Autodesk Inventor part; units mm, degrees
(part 4 of 6)
  line L1529 (-7.6457, 95.9463) -> (-7.8856, 95.9463) construction
  spline S416 degree 2 poles (-4.0547, 94.5107) (-4.2946, 94.5107) (-4.2946, 94.7506) knots 0 0 0 1 1 1
  line L1530 (-4.0547, 94.5107) -> (-4.2946, 94.5107) construction
  line L1531 (-4.2946, 94.5107) -> (-4.2946, 94.7506) construction
  spline S417 degree 2 poles (-5.0544, 95.8103) (-5.1464, 95.6784) (-5.2503, 95.6784) knots 0 0 0 1 1 1
  line L1532 (-5.0544, 95.8103) -> (-5.1464, 95.6784) construction
  line L1533 (-5.1464, 95.6784) -> (-5.2503, 95.6784) construction
  spline S418 degree 2 poles (-5.2503, 95.6784) (-5.3543, 95.6784) (-5.4463, 95.8103) knots 0 0 0 1 1 1
  line L1534 (-5.2503, 95.6784) -> (-5.3543, 95.6784) construction
  line L1535 (-5.3543, 95.6784) -> (-5.4463, 95.8103) construction
  spline S419 degree 2 poles (-6.2061, 94.7506) (-6.2061, 94.5107) (-6.446, 94.5107) knots 0 0 0 1 1 1
  line L1536 (-6.2061, 94.7506) -> (-6.2061, 94.5107) construction
  line L1537 (-6.2061, 94.5107) -> (-6.446, 94.5107) construction
  spline S420 degree 2 poles (-6.446, 94.5107) (-6.6859, 94.5107) (-6.6859, 94.7506) knots 0 0 0 1 1 1
  line L1538 (-6.446, 94.5107) -> (-6.6859, 94.5107) construction
  line L1539 (-6.6859, 94.5107) -> (-6.6859, 94.7506) construction
  line L1540 (-6.6859, 94.7506) -> (-6.6859, 97.6258)
  spline S421 degree 2 poles (-6.6859, 97.6258) (-6.6859, 97.9018) (-6.474, 97.9018) knots 0 0 0 1 1 1
  line L1541 (-6.6859, 97.6258) -> (-6.6859, 97.9018) construction
  line L1542 (-6.6859, 97.9018) -> (-6.474, 97.9018) construction
  spline S422 degree 2 poles (-6.474, 97.9018) (-6.35, 97.9018) (-6.25, 97.7618) knots 0 0 0 1 1 1
  line L1543 (-6.474, 97.9018) -> (-6.35, 97.9018) construction
  line L1544 (-6.35, 97.9018) -> (-6.25, 97.7618) construction
  spline S423 degree 2 poles (-4.2506, 97.7618) (-4.1506, 97.9018) (-4.0267, 97.9018) knots 0 0 0 1 1 1
  line L1545 (-4.2506, 97.7618) -> (-4.1506, 97.9018) construction
  line L1546 (-4.1506, 97.9018) -> (-4.0267, 97.9018) construction
  spline S424 degree 2 poles (-4.0267, 97.9018) (-3.8147, 97.9018) (-3.8147, 97.6258) knots 0 0 0 1 1 1
  line L1547 (-4.0267, 97.9018) -> (-3.8147, 97.9018) construction
  line L1548 (-3.8147, 97.9018) -> (-3.8147, 97.6258) construction
  line L1549 (-3.8147, 97.6258) -> (-3.8147, 94.7506)
  spline S425 degree 2 poles (-3.8147, 94.7506) (-3.8147, 94.5107) (-4.0547, 94.5107) knots 0 0 0 1 1 1
  line L1550 (-3.8147, 94.7506) -> (-3.8147, 94.5107) construction
  line L1551 (-3.8147, 94.5107) -> (-4.0547, 94.5107) construction
  spline S426 degree 2 poles (-0.2237, 94.5107) (-0.4637, 94.5107) (-0.4637, 94.7506) knots 0 0 0 1 1 1
  line L1552 (-0.2237, 94.5107) -> (-0.4637, 94.5107) construction
  line L1553 (-0.4637, 94.5107) -> (-0.4637, 94.7506) construction
  line L1554 (-0.4637, 94.7506) -> (-0.4637, 97.6218)
  spline S427 degree 2 poles (-0.4637, 97.6218) (-0.4637, 97.8618) (-0.2237, 97.8618) knots 0 0 0 1 1 1
  line L1555 (-0.4637, 97.6218) -> (-0.4637, 97.8618) construction
  line L1556 (-0.4637, 97.8618) -> (-0.2237, 97.8618) construction
  spline S428 degree 2 poles (-0.2237, 97.8618) (0.0162, 97.8618) (0.0162, 97.6218) knots 0 0 0 1 1 1
  line L1557 (-0.2237, 97.8618) -> (0.0162, 97.8618) construction
  line L1558 (0.0162, 97.8618) -> (0.0162, 97.6218) construction
  line L1559 (0.0162, 97.6218) -> (0.0162, 94.7506)
  spline S429 degree 2 poles (0.0162, 94.7506) (0.0162, 94.5107) (-0.2237, 94.5107) knots 0 0 0 1 1 1
  line L1560 (0.0162, 94.7506) -> (0.0162, 94.5107) construction
  line L1561 (0.0162, 94.5107) -> (-0.2237, 94.5107) construction
  spline S430 degree 2 poles (-14.794, 103.4621) (-14.4671, 103.4675) (-14.0039, 103.7345) (-13.8405, 104.1159) knots 0 0 0 1 2 2 2
  line L1562 (-14.794, 103.4621) -> (-14.4671, 103.4675) construction
  line L1563 (-14.4671, 103.4675) -> (-14.0039, 103.7345) construction
  line L1564 (-14.0039, 103.7345) -> (-13.8405, 104.1159) construction
  spline S431 degree 2 poles (-13.8405, 104.1159) (-13.7914, 104.2303) (-13.6716, 104.53) (-13.6334, 104.6444) knots 0 0 0 1 2 2 2
  line L1565 (-13.8405, 104.1159) -> (-13.7914, 104.2303) construction
  line L1566 (-13.7914, 104.2303) -> (-13.6716, 104.53) construction
  line L1567 (-13.6716, 104.53) -> (-13.6334, 104.6444) construction
  spline S432 degree 2 poles (-13.6334, 104.6444) (-13.4373, 105.2002) (-12.7344, 105.6579) (-12.1677, 105.6579) knots 0 0 0 1 2 2 2
  line L1568 (-13.6334, 104.6444) -> (-13.4373, 105.2002) construction
  line L1569 (-13.4373, 105.2002) -> (-12.7344, 105.6579) construction
  line L1570 (-12.7344, 105.6579) -> (-12.1677, 105.6579) construction
  spline S433 degree 2 poles (-12.135, 104.9278) (-12.4892, 104.9278) (-12.8434, 104.6335) (-12.9632, 104.2412) knots 0 0 0 1 2 2 2
  line L1571 (-12.135, 104.9278) -> (-12.4892, 104.9278) construction
  line L1572 (-12.4892, 104.9278) -> (-12.8434, 104.6335) construction
  line L1573 (-12.8434, 104.6335) -> (-12.9632, 104.2412) construction
  spline S434 degree 2 poles (-12.9632, 104.2412) (-13.0886, 103.8489) (-13.4318, 103.413) (-13.6389, 103.2931) knots 0 0 0 1 2 2 2
  line L1574 (-12.9632, 104.2412) -> (-13.0886, 103.8489) construction
  line L1575 (-13.0886, 103.8489) -> (-13.4318, 103.413) construction
  line L1576 (-13.4318, 103.413) -> (-13.6389, 103.2931) construction
  spline S435 degree 2 poles (21.3473, 101.4733) (21.5271, 101.5931) (21.696, 101.9092) (21.696, 102.1598) knots 0 0 0 1 2 2 2
  line L1577 (21.3473, 101.4733) -> (21.5271, 101.5931) construction
  line L1578 (21.5271, 101.5931) -> (21.696, 101.9092) construction
  line L1579 (21.696, 101.9092) -> (21.696, 102.1598) construction
  spline S436 degree 2 poles (21.696, 102.1598) (21.696, 102.3887) (21.538, 102.7374) (21.3582, 102.8463) knots 0 0 0 1 2 2 2
  line L1580 (21.696, 102.1598) -> (21.696, 102.3887) construction
  line L1581 (21.696, 102.3887) -> (21.538, 102.7374) construction
  line L1582 (21.538, 102.7374) -> (21.3582, 102.8463) construction
  spline S437 degree 2 poles (21.3582, 102.8463) (21.1675, 102.9608) (20.688, 103.0044) (20.2412, 103.0044) knots 0 0 0 1 2 2 2
  line L1583 (21.3582, 102.8463) -> (21.1675, 102.9608) construction
  line L1584 (21.1675, 102.9608) -> (20.688, 103.0044) construction
  line L1585 (20.688, 103.0044) -> (20.2412, 103.0044) construction
  spline S438 degree 2 poles (20.2194, 101.288) (20.6716, 101.288) (21.1675, 101.3643) (21.3473, 101.4733) knots 0 0 0 1 2 2 2
  line L1586 (20.2194, 101.288) -> (20.6716, 101.288) construction
  line L1587 (20.6716, 101.288) -> (21.1675, 101.3643) construction
  line L1588 (21.1675, 101.3643) -> (21.3473, 101.4733) construction
  spline S439 degree 2 poles (22.0284, 101.0265) (21.7287, 100.8031) (21.053, 100.6124) (20.5245, 100.6124) knots 0 0 0 1 2 2 2
  line L1589 (22.0284, 101.0265) -> (21.7287, 100.8031) construction
  line L1590 (21.7287, 100.8031) -> (21.053, 100.6124) construction
  line L1591 (21.053, 100.6124) -> (20.5245, 100.6124) construction
  spline S440 degree 2 poles (20.5463, 103.6909) (21.113, 103.6909) (21.7396, 103.571) (22.0502, 103.3422) knots 0 0 0 1 2 2 2
  line L1592 (20.5463, 103.6909) -> (21.113, 103.6909) construction
  line L1593 (21.113, 103.6909) -> (21.7396, 103.571) construction
  line L1594 (21.7396, 103.571) -> (22.0502, 103.3422) construction
  spline S441 degree 2 poles (22.0502, 103.3422) (22.3117, 103.1515) (22.5732, 102.5467) (22.5732, 102.1762) knots 0 0 0 1 2 2 2
  line L1595 (22.0502, 103.3422) -> (22.3117, 103.1515) construction
  line L1596 (22.3117, 103.1515) -> (22.5732, 102.5467) construction
  line L1597 (22.5732, 102.5467) -> (22.5732, 102.1762) construction
  spline S442 degree 2 poles (22.5732, 102.1762) (22.5732, 101.8111) (22.279, 101.2117) (22.0284, 101.0265) knots 0 0 0 1 2 2 2
  line L1598 (22.5732, 102.1762) -> (22.5732, 101.8111) construction
  line L1599 (22.5732, 101.8111) -> (22.279, 101.2117) construction
  line L1600 (22.279, 101.2117) -> (22.0284, 101.0265) construction
  spline S443 degree 2 poles (-15.4296, 28.4883) (-15.4296, 28.5843) (-15.2856, 28.7283) (-15.1896, 28.7283) knots 0 0 0 1 2 2 2
  line L1601 (-15.4296, 28.4883) -> (-15.4296, 28.5843) construction
  line L1602 (-15.4296, 28.5843) -> (-15.2856, 28.7283) construction
  line L1603 (-15.2856, 28.7283) -> (-15.1896, 28.7283) construction
  line L1604 (-15.1896, 28.7283) -> (-13.994, 28.7283)
  spline S444 degree 2 poles (-11.0308, 28.5323) (-10.6469, 28.7283) (-10.163, 28.7283) knots 0 0 0 1 1 1
  line L1605 (-11.0308, 28.5323) -> (-10.6469, 28.7283) construction
  line L1606 (-10.6469, 28.7283) -> (-10.163, 28.7283) construction
  spline S445 degree 2 poles (-10.163, 28.7283) (-9.4432, 28.7283) (-8.8754, 28.3244) knots 0 0 0 1 1 1
  line L1607 (-10.163, 28.7283) -> (-9.4432, 28.7283) construction
  line L1608 (-9.4432, 28.7283) -> (-8.8754, 28.3244) construction
  spline S446 degree 2 poles (-3.0595, 28.1573) (-3.0595, 27.9163) (-3.3004, 27.9163) knots 0 0 0 1 1 1
  line L1609 (-3.0595, 28.1573) -> (-3.0595, 27.9163) construction
  line L1610 (-3.0595, 27.9163) -> (-3.3004, 27.9163) construction
  spline S447 degree 2 poles (-3.3004, 27.9163) (-3.5413, 27.9163) (-3.5413, 28.1573) knots 0 0 0 1 1 1
  line L1611 (-3.3004, 27.9163) -> (-3.5413, 27.9163) construction
  line L1612 (-3.5413, 27.9163) -> (-3.5413, 28.1573) construction
  line L1613 (0.2406, 29.0322) -> (-0.1335, 29.0322)
  spline S448 degree 2 poles (1.1789, 29.029) (1.125, 29.029) (1.0585, 29.0576) knots 0 0 0 1 1 1
  line L1614 (1.1789, 29.029) -> (1.125, 29.029) construction
  line L1615 (1.125, 29.029) -> (1.0585, 29.0576) construction
  spline S449 degree 2 poles (1.7464, 32.4495) (1.6639, 32.532) (1.6639, 32.6397) knots 0 0 0 1 1 1
  line L1616 (1.7464, 32.4495) -> (1.6639, 32.532) construction
  line L1617 (1.6639, 32.532) -> (1.6639, 32.6397) construction
  spline S450 degree 2 poles (1.6639, 32.6397) (1.6639, 32.8616) (1.9144, 32.8616) knots 0 0 0 1 1 1
  line L1618 (1.6639, 32.6397) -> (1.6639, 32.8616) construction
  line L1619 (1.6639, 32.8616) -> (1.9144, 32.8616) construction
  line L1620 (12.7332, 29.0126) -> (12.1753, 29.0126)
  spline S451 degree 2 poles (18.1952, 28.6956) (18.1952, 28.3627) (17.7261, 27.8967) (17.3932, 27.8967) knots 0 0 0 1 2 2 2
  line L1621 (18.1952, 28.6956) -> (18.1952, 28.3627) construction
  line L1622 (18.1952, 28.3627) -> (17.7261, 27.8967) construction
  line L1623 (17.7261, 27.8967) -> (17.3932, 27.8967) construction
  line L1624 (17.3932, 27.8967) -> (16.6451, 27.8967)
  spline S452 degree 2 poles (16.6451, 27.8967) (16.4041, 27.8967) (16.4041, 28.1377) knots 0 0 0 1 1 1
  line L1625 (16.6451, 27.8967) -> (16.4041, 27.8967) construction
  line L1626 (16.4041, 27.8967) -> (16.4041, 28.1377) construction
  spline S453 degree 2 poles (16.4041, 28.1377) (16.4041, 28.3754) (16.6451, 28.3754) knots 0 0 0 1 1 1
  line L1627 (16.4041, 28.1377) -> (16.4041, 28.3754) construction
  line L1628 (16.4041, 28.3754) -> (16.6451, 28.3754) construction
  line L1629 (16.6451, 28.3754) -> (17.3932, 28.3754)
  spline S454 degree 2 poles (17.3932, 28.3754) (17.5232, 28.3754) (17.7134, 28.5656) (17.7134, 28.6956) knots 0 0 0 1 2 2 2
  line L1630 (17.3932, 28.3754) -> (17.5232, 28.3754) construction
  line L1631 (17.5232, 28.3754) -> (17.7134, 28.5656) construction
  line L1632 (17.7134, 28.5656) -> (17.7134, 28.6956) construction
  spline S455 degree 2 poles (-16.9273, 1.4084) (-16.7313, 1.4084) (-16.4514, 1.6923) (-16.4514, 1.8882) knots 0 0 0 1 2 2 2
  line L1633 (-16.9273, 1.4084) -> (-16.7313, 1.4084) construction
  line L1634 (-16.7313, 1.4084) -> (-16.4514, 1.6923) construction
  line L1635 (-16.4514, 1.6923) -> (-16.4514, 1.8882) construction
  spline S456 degree 2 poles (-17.4071, 3.7997) (-17.6031, 3.7997) (-17.883, 3.5158) (-17.883, 3.3198) knots 0 0 0 1 2 2 2
  line L1636 (-17.4071, 3.7997) -> (-17.6031, 3.7997) construction
  line L1637 (-17.6031, 3.7997) -> (-17.883, 3.5158) construction
  line L1638 (-17.883, 3.5158) -> (-17.883, 3.3198) construction
  line L1639 (-17.883, 3.3198) -> (-17.883, 1.8882)
  spline S457 degree 2 poles (-17.883, 1.8882) (-17.883, 1.6923) (-17.6031, 1.4084) (-17.4071, 1.4084) knots 0 0 0 1 2 2 2
  line L1640 (-17.883, 1.8882) -> (-17.883, 1.6923) construction
  line L1641 (-17.883, 1.6923) -> (-17.6031, 1.4084) construction
  line L1642 (-17.6031, 1.4084) -> (-17.4071, 1.4084) construction
  line L1643 (-17.4071, 1.4084) -> (-16.9273, 1.4084)
  line L1644 (-16.9273, 0.9285) -> (-17.4071, 0.9285)
  spline S458 degree 2 poles (-17.4071, 0.9285) (-17.799, 0.9285) (-18.3629, 1.4884) (-18.3629, 1.8842) knots 0 0 0 1 2 2 2
  line L1645 (-17.4071, 0.9285) -> (-17.799, 0.9285) construction
  line L1646 (-17.799, 0.9285) -> (-18.3629, 1.4884) construction
  line L1647 (-18.3629, 1.4884) -> (-18.3629, 1.8842) construction
  line L1648 (-18.3629, 1.8842) -> (-18.3629, 3.3238)
  spline S459 degree 2 poles (-18.3629, 3.3238) (-18.3629, 3.7197) (-17.799, 4.2796) (-17.4071, 4.2796) knots 0 0 0 1 2 2 2
  line L1649 (-18.3629, 3.3238) -> (-18.3629, 3.7197) construction
  line L1650 (-18.3629, 3.7197) -> (-17.799, 4.2796) construction
  line L1651 (-17.799, 4.2796) -> (-17.4071, 4.2796) construction
  line L1652 (-17.4071, 4.2796) -> (-16.2115, 4.2796)
  spline S460 degree 2 poles (-16.2115, 4.2796) (-15.9715, 4.2796) (-15.9715, 4.0396) knots 0 0 0 1 1 1
  line L1653 (-16.2115, 4.2796) -> (-15.9715, 4.2796) construction
  line L1654 (-15.9715, 4.2796) -> (-15.9715, 4.0396) construction
  line L1655 (-15.9715, 4.0396) -> (-15.9715, 1.8922)
  spline S461 degree 2 poles (-15.9715, 1.8922) (-15.9715, 1.5323) (-15.6356, 1.3884) knots 0 0 0 1 1 1
  line L1656 (-15.9715, 1.8922) -> (-15.9715, 1.5323) construction
  line L1657 (-15.9715, 1.5323) -> (-15.6356, 1.3884) construction
  spline S462 degree 2 poles (-15.6356, 1.3884) (-15.4877, 1.3284) (-15.4877, 1.1764) knots 0 0 0 1 1 1
  line L1658 (-15.6356, 1.3884) -> (-15.4877, 1.3284) construction
  line L1659 (-15.4877, 1.3284) -> (-15.4877, 1.1764) construction
  spline S463 degree 2 poles (-15.4877, 1.1764) (-15.4877, 1.0765) (-15.6236, 0.9245) (-15.7236, 0.9245) knots 0 0 0 1 2 2 2
  line L1660 (-15.4877, 1.1764) -> (-15.4877, 1.0765) construction
  line L1661 (-15.4877, 1.0765) -> (-15.6236, 0.9245) construction
  line L1662 (-15.6236, 0.9245) -> (-15.7236, 0.9245) construction
  spline S464 degree 2 poles (-15.7236, 0.9245) (-15.7756, 0.9245) (-15.8276, 0.9485) knots 0 0 0 1 1 1
  line L1663 (-15.7236, 0.9245) -> (-15.7756, 0.9245) construction
  line L1664 (-15.7756, 0.9245) -> (-15.8276, 0.9485) construction
  spline S465 degree 2 poles (-15.8276, 0.9485) (-16.0675, 1.0525) (-16.2155, 1.2444) knots 0 0 0 1 1 1
  line L1665 (-15.8276, 0.9485) -> (-16.0675, 1.0525) construction
  line L1666 (-16.0675, 1.0525) -> (-16.2155, 1.2444) construction
  spline S466 degree 2 poles (-16.2155, 1.2444) (-16.5034, 0.9285) (-16.9273, 0.9285) knots 0 0 0 1 1 1
  line L1667 (-16.2155, 1.2444) -> (-16.5034, 0.9285) construction
  line L1668 (-16.5034, 0.9285) -> (-16.9273, 0.9285) construction
  spline S467 degree 2 poles (-12.8604, 0.9285) (-13.1003, 0.9285) (-13.1003, 1.1685) knots 0 0 0 1 1 1
  line L1669 (-12.8604, 0.9285) -> (-13.1003, 0.9285) construction
  line L1670 (-13.1003, 0.9285) -> (-13.1003, 1.1685) construction
  line L1671 (-13.1003, 1.1685) -> (-13.1003, 3.3198)
  spline S468 degree 2 poles (-13.1003, 3.3198) (-13.1003, 3.5158) (-13.3803, 3.7997) (-13.5762, 3.7997) knots 0 0 0 1 2 2 2
  line L1672 (-13.1003, 3.3198) -> (-13.1003, 3.5158) construction
  line L1673 (-13.1003, 3.5158) -> (-13.3803, 3.7997) construction
  line L1674 (-13.3803, 3.7997) -> (-13.5762, 3.7997) construction
  spline S469 degree 2 poles (-14.5319, 1.1685) (-14.5319, 0.9285) (-14.7719, 0.9285) knots 0 0 0 1 1 1
  line L1675 (-14.5319, 1.1685) -> (-14.5319, 0.9285) construction
  line L1676 (-14.5319, 0.9285) -> (-14.7719, 0.9285) construction
  spline S470 degree 2 poles (-14.7719, 0.9285) (-15.0118, 0.9285) (-15.0118, 1.1685) knots 0 0 0 1 1 1
  line L1677 (-14.7719, 0.9285) -> (-15.0118, 0.9285) construction
  line L1678 (-15.0118, 0.9285) -> (-15.0118, 1.1685) construction
  line L1679 (-15.0118, 1.1685) -> (-15.0118, 4.0396)
  spline S471 degree 2 poles (-15.0118, 4.0396) (-15.0118, 4.2796) (-14.7719, 4.2796) knots 0 0 0 1 1 1
  line L1680 (-15.0118, 4.0396) -> (-15.0118, 4.2796) construction
  line L1681 (-15.0118, 4.2796) -> (-14.7719, 4.2796) construction
  line L1682 (-14.7719, 4.2796) -> (-13.5762, 4.2796)
  spline S472 degree 2 poles (-13.5762, 4.2796) (-13.1803, 4.2796) (-12.6205, 3.7197) (-12.6205, 3.3238) knots 0 0 0 1 2 2 2
  line L1683 (-13.5762, 4.2796) -> (-13.1803, 4.2796) construction
  line L1684 (-13.1803, 4.2796) -> (-12.6205, 3.7197) construction
  line L1685 (-12.6205, 3.7197) -> (-12.6205, 3.3238) construction
  line L1686 (-12.6205, 3.3238) -> (-12.6205, 1.1685)
  spline S473 degree 2 poles (-12.6205, 1.1685) (-12.6205, 0.9285) (-12.8604, 0.9285) knots 0 0 0 1 1 1
  line L1687 (-12.6205, 1.1685) -> (-12.6205, 0.9285) construction
  line L1688 (-12.6205, 0.9285) -> (-12.8604, 0.9285) construction
  spline S474 degree 2 poles (-15.1075, 7.2002) (-15.2434, 7.2002) (-15.3154, 7.3282) knots 0 0 0 1 1 1
  line L1689 (-15.1075, 7.2002) -> (-15.2434, 7.2002) construction
  line L1690 (-15.2434, 7.2002) -> (-15.3154, 7.3282) construction
  spline S475 degree 2 poles (-17.2869, 7.4441) (-17.2869, 7.2042) (-17.5268, 7.2042) knots 0 0 0 1 1 1
  line L1691 (-17.2869, 7.4441) -> (-17.2869, 7.2042) construction
  line L1692 (-17.2869, 7.2042) -> (-17.5268, 7.2042) construction
  spline S476 degree 2 poles (-17.5268, 7.2042) (-17.7667, 7.2042) (-17.7667, 7.4441) knots 0 0 0 1 1 1
  line L1693 (-17.5268, 7.2042) -> (-17.7667, 7.2042) construction
  line L1694 (-17.7667, 7.2042) -> (-17.7667, 7.4441) construction
  line L1695 (-17.7667, 7.4441) -> (-17.7667, 11.7509)
  spline S477 degree 2 poles (-17.7667, 11.7509) (-17.7667, 11.9869) (-17.5268, 11.9869) knots 0 0 0 1 1 1
  line L1696 (-17.7667, 11.7509) -> (-17.7667, 11.9869) construction
  line L1697 (-17.7667, 11.9869) -> (-17.5268, 11.9869) construction
  spline S478 degree 2 poles (-17.5268, 11.9869) (-17.2869, 11.9869) (-17.2869, 11.7509) knots 0 0 0 1 1 1
  line L1698 (-17.5268, 11.9869) -> (-17.2869, 11.9869) construction
  line L1699 (-17.2869, 11.9869) -> (-17.2869, 11.7509) construction
  spline S479 degree 2 poles (-15.2714, 11.9189) (-15.1995, 11.9909) (-15.1075, 11.9909) knots 0 0 0 1 1 1
  line L1700 (-15.2714, 11.9189) -> (-15.1995, 11.9909) construction
  line L1701 (-15.1995, 11.9909) -> (-15.1075, 11.9909) construction
  spline S480 degree 2 poles (-15.1075, 11.9909) (-15.0115, 11.9909) (-14.8635, 11.8429) (-14.8635, 11.7469) knots 0 0 0 1 2 2 2
  line L1702 (-15.1075, 11.9909) -> (-15.0115, 11.9909) construction
  line L1703 (-15.0115, 11.9909) -> (-14.8635, 11.8429) construction
  line L1704 (-14.8635, 11.8429) -> (-14.8635, 11.7469) construction
  spline S481 degree 2 poles (-14.8635, 11.7469) (-14.8635, 11.6549) (-14.9355, 11.583) knots 0 0 0 1 1 1
  line L1705 (-14.8635, 11.7469) -> (-14.8635, 11.6549) construction
  line L1706 (-14.8635, 11.6549) -> (-14.9355, 11.583) construction
  spline S482 degree 2 poles (-14.8915, 7.5601) (-14.8595, 7.4961) (-14.8595, 7.4361) knots 0 0 0 1 1 1
  line L1707 (-14.8915, 7.5601) -> (-14.8595, 7.4961) construction
  line L1708 (-14.8595, 7.4961) -> (-14.8595, 7.4361) construction
  spline S483 degree 2 poles (-14.8595, 7.4361) (-14.8595, 7.3402) (-15.0115, 7.2002) (-15.1075, 7.2002) knots 0 0 0 1 2 2 2
  line L1709 (-14.8595, 7.4361) -> (-14.8595, 7.3402) construction
  line L1710 (-14.8595, 7.3402) -> (-15.0115, 7.2002) construction
  line L1711 (-15.0115, 7.2002) -> (-15.1075, 7.2002) construction
  spline S484 degree 2 poles (-17.3876, -9.5445) (-17.8875, -9.5445) (-18.5873, -8.8447) (-18.5873, -8.3488) knots 0 0 0 1 2 2 2
  line L1712 (-17.3876, -9.5445) -> (-17.8875, -9.5445) construction
  line L1713 (-17.8875, -9.5445) -> (-18.5873, -8.8447) construction
  line L1714 (-18.5873, -8.8447) -> (-18.5873, -8.3488) construction
  line L1715 (-18.5873, -8.3488) -> (-18.5873, -5.9535)
  spline S485 degree 2 poles (-18.5873, -5.9535) (-18.5873, -5.4616) (-17.8875, -4.7578) (-17.3876, -4.7578) knots 0 0 0 1 2 2 2
  line L1716 (-18.5873, -5.9535) -> (-18.5873, -5.4616) construction
  line L1717 (-18.5873, -5.4616) -> (-17.8875, -4.7578) construction
  line L1718 (-17.8875, -4.7578) -> (-17.3876, -4.7578) construction
  line L1719 (-17.3876, -4.7578) -> (-16.4319, -4.7578)
  spline S486 degree 2 poles (-16.4319, -4.7578) (-16.1919, -4.7578) (-16.1919, -4.9978) knots 0 0 0 1 1 1
  line L1720 (-16.4319, -4.7578) -> (-16.1919, -4.7578) construction
  line L1721 (-16.1919, -4.7578) -> (-16.1919, -4.9978) construction
  spline S487 degree 2 poles (-16.1919, -4.9978) (-16.1919, -5.2377) (-16.4319, -5.2377) knots 0 0 0 1 1 1
  line L1722 (-16.1919, -4.9978) -> (-16.1919, -5.2377) construction
  line L1723 (-16.1919, -5.2377) -> (-16.4319, -5.2377) construction
  line L1724 (-16.4319, -5.2377) -> (-17.3876, -5.2377)
  spline S488 degree 2 poles (-17.3876, -5.2377) (-17.6875, -5.2377) (-18.1074, -5.6576) (-18.1074, -5.9535) knots 0 0 0 1 2 2 2
  line L1725 (-17.3876, -5.2377) -> (-17.6875, -5.2377) construction
  line L1726 (-17.6875, -5.2377) -> (-18.1074, -5.6576) construction
  line L1727 (-18.1074, -5.6576) -> (-18.1074, -5.9535) construction
  line L1728 (-18.1074, -5.9535) -> (-18.1074, -8.3488)
  spline S489 degree 2 poles (-18.1074, -8.3488) (-18.1074, -8.6447) (-17.6875, -9.0646) (-17.3876, -9.0646) knots 0 0 0 1 2 2 2
  line L1729 (-18.1074, -8.3488) -> (-18.1074, -8.6447) construction
  line L1730 (-18.1074, -8.6447) -> (-17.6875, -9.0646) construction
  line L1731 (-17.6875, -9.0646) -> (-17.3876, -9.0646) construction
  line L1732 (-17.3876, -9.0646) -> (-16.4319, -9.0646)
  spline S490 degree 2 poles (-16.4319, -9.0646) (-16.1919, -9.0646) (-16.1919, -9.3045) knots 0 0 0 1 1 1
  line L1733 (-16.4319, -9.0646) -> (-16.1919, -9.0646) construction
  line L1734 (-16.1919, -9.0646) -> (-16.1919, -9.3045) construction
  spline S491 degree 2 poles (-16.1919, -9.3045) (-16.1919, -9.5445) (-16.4319, -9.5445) knots 0 0 0 1 1 1
  line L1735 (-16.1919, -9.3045) -> (-16.1919, -9.5445) construction
  line L1736 (-16.1919, -9.5445) -> (-16.4319, -9.5445) construction
  line L1737 (-16.4319, -9.5445) -> (-17.3876, -9.5445)
  spline S492 degree 2 poles (-8.774, -9.5445) (-9.014, -9.5445) (-9.014, -9.3045) knots 0 0 0 1 1 1
  line L1738 (-8.774, -9.5445) -> (-9.014, -9.5445) construction
  line L1739 (-9.014, -9.5445) -> (-9.014, -9.3045) construction
  spline S493 degree 2 poles (-10.9254, -9.3045) (-10.9254, -9.5445) (-11.1653, -9.5445) knots 0 0 0 1 1 1
  line L1740 (-10.9254, -9.3045) -> (-10.9254, -9.5445) construction
  line L1741 (-10.9254, -9.5445) -> (-11.1653, -9.5445) construction
  spline S494 degree 2 poles (-11.1653, -9.5445) (-11.4053, -9.5445) (-11.4053, -9.3045) knots 0 0 0 1 1 1
  line L1742 (-11.1653, -9.5445) -> (-11.4053, -9.5445) construction
  line L1743 (-11.4053, -9.5445) -> (-11.4053, -9.3045) construction
  line L1744 (-11.4053, -9.3045) -> (-11.4053, -4.9978)
  spline S495 degree 2 poles (-11.4053, -4.9978) (-11.4053, -4.7578) (-11.1653, -4.7578) knots 0 0 0 1 1 1
  line L1745 (-11.4053, -4.9978) -> (-11.4053, -4.7578) construction
  line L1746 (-11.4053, -4.7578) -> (-11.1653, -4.7578) construction
  line L1747 (-11.1653, -4.7578) -> (-8.774, -4.7578)
  spline S496 degree 2 poles (-8.774, -4.7578) (-8.5341, -4.7578) (-8.5341, -4.9978) knots 0 0 0 1 1 1
  line L1748 (-8.774, -4.7578) -> (-8.5341, -4.7578) construction
  line L1749 (-8.5341, -4.7578) -> (-8.5341, -4.9978) construction
  line L1750 (-8.5341, -4.9978) -> (-8.5341, -9.3045)
  spline S497 degree 2 poles (-8.5341, -9.3045) (-8.5341, -9.5445) (-8.774, -9.5445) knots 0 0 0 1 1 1
  line L1751 (-8.5341, -9.3045) -> (-8.5341, -9.5445) construction
  line L1752 (-8.5341, -9.5445) -> (-8.774, -9.5445) construction
  spline S498 degree 2 poles (11.2339, 1.5425) (11.4299, 1.5425) (11.7098, 1.8264) (11.7098, 2.0224) knots 0 0 0 1 2 2 2
  line L1753 (11.2339, 1.5425) -> (11.4299, 1.5425) construction
  line L1754 (11.4299, 1.5425) -> (11.7098, 1.8264) construction
  line L1755 (11.7098, 1.8264) -> (11.7098, 2.0224) construction
  spline S499 degree 2 poles (10.7541, 3.9338) (10.5581, 3.9338) (10.2782, 3.6499) (10.2782, 3.454) knots 0 0 0 1 2 2 2
  line L1756 (10.7541, 3.9338) -> (10.5581, 3.9338) construction
  line L1757 (10.5581, 3.9338) -> (10.2782, 3.6499) construction
  line L1758 (10.2782, 3.6499) -> (10.2782, 3.454) construction
  line L1759 (10.2782, 3.454) -> (10.2782, 2.0224)
  spline S500 degree 2 poles (10.2782, 2.0224) (10.2782, 1.8264) (10.5581, 1.5425) (10.7541, 1.5425) knots 0 0 0 1 2 2 2
  line L1760 (10.2782, 2.0224) -> (10.2782, 1.8264) construction
  line L1761 (10.2782, 1.8264) -> (10.5581, 1.5425) construction
  line L1762 (10.5581, 1.5425) -> (10.7541, 1.5425) construction
  line L1763 (10.7541, 1.5425) -> (11.2339, 1.5425)
  line L1764 (11.2339, 1.0626) -> (10.7541, 1.0626)
  spline S501 degree 2 poles (10.7541, 1.0626) (10.3622, 1.0626) (9.7984, 1.6225) (9.7984, 2.0184) knots 0 0 0 1 2 2 2
  line L1765 (10.7541, 1.0626) -> (10.3622, 1.0626) construction
  line L1766 (10.3622, 1.0626) -> (9.7984, 1.6225) construction
  line L1767 (9.7984, 1.6225) -> (9.7984, 2.0184) construction
  line L1768 (9.7984, 2.0184) -> (9.7984, 3.458)
  spline S502 degree 2 poles (9.7984, 3.458) (9.7984, 3.8539) (10.3622, 4.4137) (10.7541, 4.4137) knots 0 0 0 1 2 2 2
  line L1769 (9.7984, 3.458) -> (9.7984, 3.8539) construction
  line L1770 (9.7984, 3.8539) -> (10.3622, 4.4137) construction
  line L1771 (10.3622, 4.4137) -> (10.7541, 4.4137) construction
  line L1772 (10.7541, 4.4137) -> (11.9497, 4.4137)
  spline S503 degree 2 poles (11.9497, 4.4137) (12.1897, 4.4137) (12.1897, 4.1738) knots 0 0 0 1 1 1
  line L1773 (11.9497, 4.4137) -> (12.1897, 4.4137) construction
  line L1774 (12.1897, 4.4137) -> (12.1897, 4.1738) construction
  line L1775 (12.1897, 4.1738) -> (12.1897, 2.0264)
  spline S504 degree 2 poles (12.1897, 2.0264) (12.1897, 1.6665) (12.5256, 1.5225) knots 0 0 0 1 1 1
  line L1776 (12.1897, 2.0264) -> (12.1897, 1.6665) construction
  line L1777 (12.1897, 1.6665) -> (12.5256, 1.5225) construction
  spline S505 degree 2 poles (12.5256, 1.5225) (12.6735, 1.4625) (12.6735, 1.3106) knots 0 0 0 1 1 1
  line L1778 (12.5256, 1.5225) -> (12.6735, 1.4625) construction
  line L1779 (12.6735, 1.4625) -> (12.6735, 1.3106) construction
  spline S506 degree 2 poles (12.6735, 1.3106) (12.6735, 1.2106) (12.5376, 1.0586) (12.4376, 1.0586) knots 0 0 0 1 2 2 2
  line L1780 (12.6735, 1.3106) -> (12.6735, 1.2106) construction
  line L1781 (12.6735, 1.2106) -> (12.5376, 1.0586) construction
  line L1782 (12.5376, 1.0586) -> (12.4376, 1.0586) construction
  spline S507 degree 2 poles (12.4376, 1.0586) (12.3856, 1.0586) (12.3336, 1.0826) knots 0 0 0 1 1 1
  line L1783 (12.4376, 1.0586) -> (12.3856, 1.0586) construction
  line L1784 (12.3856, 1.0586) -> (12.3336, 1.0826) construction
  spline S508 degree 2 poles (12.3336, 1.0826) (12.0937, 1.1866) (11.9457, 1.3786) knots 0 0 0 1 1 1
  line L1785 (12.3336, 1.0826) -> (12.0937, 1.1866) construction
  line L1786 (12.0937, 1.1866) -> (11.9457, 1.3786) construction
  spline S509 degree 2 poles (11.9457, 1.3786) (11.6578, 1.0626) (11.2339, 1.0626) knots 0 0 0 1 1 1
  line L1787 (11.9457, 1.3786) -> (11.6578, 1.0626) construction
  line L1788 (11.6578, 1.0626) -> (11.2339, 1.0626) construction
  spline S510 degree 2 poles (14.585, 1.5425) (14.7809, 1.5425) (15.0609, 1.8264) (15.0609, 2.0224) knots 0 0 0 1 2 2 2
  line L1789 (14.585, 1.5425) -> (14.7809, 1.5425) construction
  line L1790 (14.7809, 1.5425) -> (15.0609, 1.8264) construction
  line L1791 (15.0609, 1.8264) -> (15.0609, 2.0224) construction
  line L1792 (15.0609, 2.0224) -> (15.0609, 3.454)
  spline S511 degree 2 poles (15.0609, 3.454) (15.0609, 3.6499) (14.7809, 3.9338) (14.585, 3.9338) knots 0 0 0 1 2 2 2
  line L1793 (15.0609, 3.454) -> (15.0609, 3.6499) construction
  line L1794 (15.0609, 3.6499) -> (14.7809, 3.9338) construction
  line L1795 (14.7809, 3.9338) -> (14.585, 3.9338) construction
  spline S512 degree 2 poles (13.6293, -0.133) (13.6293, -0.3729) (13.3893, -0.3729) knots 0 0 0 1 1 1
  line L1796 (13.6293, -0.133) -> (13.6293, -0.3729) construction
  line L1797 (13.6293, -0.3729) -> (13.3893, -0.3729) construction
  spline S513 degree 2 poles (13.3893, -0.3729) (13.1494, -0.3729) (13.1494, -0.133) knots 0 0 0 1 1 1
  line L1798 (13.3893, -0.3729) -> (13.1494, -0.3729) construction
  line L1799 (13.1494, -0.3729) -> (13.1494, -0.133) construction
  line L1800 (13.1494, -0.133) -> (13.1494, 4.1738)
  spline S514 degree 2 poles (13.1494, 4.1738) (13.1494, 4.4137) (13.3893, 4.4137) knots 0 0 0 1 1 1
  line L1801 (13.1494, 4.1738) -> (13.1494, 4.4137) construction
  line L1802 (13.1494, 4.4137) -> (13.3893, 4.4137) construction
  line L1803 (13.3893, 4.4137) -> (14.585, 4.4137)
  spline S515 degree 2 poles (14.585, 4.4137) (14.9809, 4.4137) (15.5407, 3.8539) (15.5407, 3.458) knots 0 0 0 1 2 2 2
  line L1804 (14.585, 4.4137) -> (14.9809, 4.4137) construction
  line L1805 (14.9809, 4.4137) -> (15.5407, 3.8539) construction
  line L1806 (15.5407, 3.8539) -> (15.5407, 3.458) construction
  line L1807 (15.5407, 3.458) -> (15.5407, 2.0184)
  spline S516 degree 2 poles (15.5407, 2.0184) (15.5407, 1.6225) (14.9809, 1.0626) (14.585, 1.0626) knots 0 0 0 1 2 2 2
  line L1808 (15.5407, 2.0184) -> (15.5407, 1.6225) construction
  line L1809 (15.5407, 1.6225) -> (14.9809, 1.0626) construction
  line L1810 (14.9809, 1.0626) -> (14.585, 1.0626) construction
  spline S517 degree 2 poles (3.0435, -7.2929) (2.8035, -7.2929) (2.8035, -7.053) knots 0 0 0 1 1 1
  line L1811 (3.0435, -7.2929) -> (2.8035, -7.2929) construction
  line L1812 (2.8035, -7.2929) -> (2.8035, -7.053) construction
  spline S518 degree 2 poles (2.8035, -7.053) (2.8035, -6.8131) (3.0435, -6.8131) knots 0 0 0 1 1 1
  line L1813 (2.8035, -7.053) -> (2.8035, -6.8131) construction
  line L1814 (2.8035, -6.8131) -> (3.0435, -6.8131) construction
  line L1815 (3.0435, -6.8131) -> (3.2834, -6.8131)
  spline S519 degree 2 poles (3.2834, -6.8131) (3.5073, -6.8131) (3.6393, -6.6651) knots 0 0 0 1 1 1
  line L1816 (3.2834, -6.8131) -> (3.5073, -6.8131) construction
  line L1817 (3.5073, -6.8131) -> (3.6393, -6.6651) construction
  spline S520 degree 2 poles (3.6393, -6.6651) (3.7593, -6.5291) (3.7593, -6.3332) knots 0 0 0 1 1 1
  line L1818 (3.6393, -6.6651) -> (3.7593, -6.5291) construction
  line L1819 (3.7593, -6.5291) -> (3.7593, -6.3332) construction
  spline S521 degree 2 poles (3.7593, -6.3332) (3.7593, -6.1373) (3.6393, -6.0053) knots 0 0 0 1 1 1
  line L1820 (3.7593, -6.3332) -> (3.7593, -6.1373) construction
  line L1821 (3.7593, -6.1373) -> (3.6393, -6.0053) construction
  spline S522 degree 2 poles (3.6393, -6.0053) (3.5073, -5.8573) (3.2794, -5.8573) knots 0 0 0 1 1 1
  line L1822 (3.6393, -6.0053) -> (3.5073, -5.8573) construction
  line L1823 (3.5073, -5.8573) -> (3.2794, -5.8573) construction
  line L1824 (3.2794, -5.8573) -> (3.0395, -5.8573)
  spline S523 degree 2 poles (3.0395, -5.8573) (2.7156, -5.8573) (2.4676, -6.0493) knots 0 0 0 1 1 1
  line L1825 (3.0395, -5.8573) -> (2.7156, -5.8573) construction
  line L1826 (2.7156, -5.8573) -> (2.4676, -6.0493) construction
  spline S524 degree 2 poles (2.4676, -6.0493) (2.3957, -6.1013) (2.3197, -6.1013) knots 0 0 0 1 1 1
  line L1827 (2.4676, -6.0493) -> (2.3957, -6.1013) construction
  line L1828 (2.3957, -6.1013) -> (2.3197, -6.1013) construction
  spline S525 degree 2 poles (2.3197, -6.1013) (2.2237, -6.1013) (2.0797, -5.9533) (2.0797, -5.8533) knots 0 0 0 1 2 2 2
  line L1829 (2.3197, -6.1013) -> (2.2237, -6.1013) construction
  line L1830 (2.2237, -6.1013) -> (2.0797, -5.9533) construction
  line L1831 (2.0797, -5.9533) -> (2.0797, -5.8533) construction
  spline S526 degree 2 poles (2.0797, -5.8533) (2.0797, -5.7414) (2.1797, -5.6654) knots 0 0 0 1 1 1
  line L1832 (2.0797, -5.8533) -> (2.0797, -5.7414) construction
  line L1833 (2.0797, -5.7414) -> (2.1797, -5.6654) construction
  spline S527 degree 2 poles (2.1797, -5.6654) (2.5516, -5.3775) (3.0395, -5.3775) knots 0 0 0 1 1 1
  line L1834 (2.1797, -5.6654) -> (2.5516, -5.3775) construction
  line L1835 (2.5516, -5.3775) -> (3.0395, -5.3775) construction
  line L1836 (3.0395, -5.3775) -> (3.2794, -5.3775)
  spline S528 degree 2 poles (3.2794, -5.3775) (3.7313, -5.3775) (3.9992, -5.6734) knots 0 0 0 1 1 1
  line L1837 (3.2794, -5.3775) -> (3.7313, -5.3775) construction
  line L1838 (3.7313, -5.3775) -> (3.9992, -5.6734) construction
  spline S529 degree 2 poles (3.9992, -5.6734) (4.2391, -5.9453) (4.2391, -6.3332) knots 0 0 0 1 1 1
  line L1839 (3.9992, -5.6734) -> (4.2391, -5.9453) construction
  line L1840 (4.2391, -5.9453) -> (4.2391, -6.3332) construction
  spline S530 degree 2 poles (4.2391, -6.3332) (4.2391, -6.7771) (3.9392, -7.053) knots 0 0 0 1 1 1
  line L1841 (4.2391, -6.3332) -> (4.2391, -6.7771) construction
  line L1842 (4.2391, -6.7771) -> (3.9392, -7.053) construction
  spline S531 degree 2 poles (3.9392, -7.053) (4.2391, -7.3289) (4.2391, -7.7728) knots 0 0 0 1 1 1
  line L1843 (3.9392, -7.053) -> (4.2391, -7.3289) construction
  line L1844 (4.2391, -7.3289) -> (4.2391, -7.7728) construction
  spline S532 degree 2 poles (4.2391, -7.7728) (4.2391, -8.1647) (3.9992, -8.4326) knots 0 0 0 1 1 1
  line L1845 (4.2391, -7.7728) -> (4.2391, -8.1647) construction
  line L1846 (4.2391, -8.1647) -> (3.9992, -8.4326) construction
  spline S533 degree 2 poles (3.9992, -8.4326) (3.7313, -8.7285) (3.2794, -8.7285) knots 0 0 0 1 1 1
  line L1847 (3.9992, -8.4326) -> (3.7313, -8.7285) construction
  line L1848 (3.7313, -8.7285) -> (3.2794, -8.7285) construction
  line L1849 (3.2794, -8.7285) -> (3.0395, -8.7285)
  spline S534 degree 2 poles (3.0395, -8.7285) (2.5516, -8.7285) (2.1797, -8.4406) knots 0 0 0 1 1 1
  line L1850 (3.0395, -8.7285) -> (2.5516, -8.7285) construction
  line L1851 (2.5516, -8.7285) -> (2.1797, -8.4406) construction
  spline S535 degree 2 poles (2.1797, -8.4406) (2.0797, -8.3646) (2.0797, -8.2527) knots 0 0 0 1 1 1
  line L1852 (2.1797, -8.4406) -> (2.0797, -8.3646) construction
  line L1853 (2.0797, -8.3646) -> (2.0797, -8.2527) construction
  spline S536 degree 2 poles (2.0797, -8.2527) (2.0797, -8.1527) (2.2237, -8.0047) (2.3197, -8.0047) knots 0 0 0 1 2 2 2
  line L1854 (2.0797, -8.2527) -> (2.0797, -8.1527) construction
  line L1855 (2.0797, -8.1527) -> (2.2237, -8.0047) construction
  line L1856 (2.2237, -8.0047) -> (2.3197, -8.0047) construction
  spline S537 degree 2 poles (2.3197, -8.0047) (2.3957, -8.0047) (2.4676, -8.0567) knots 0 0 0 1 1 1
  line L1857 (2.3197, -8.0047) -> (2.3957, -8.0047) construction
  line L1858 (2.3957, -8.0047) -> (2.4676, -8.0567) construction
  spline S538 degree 2 poles (2.4676, -8.0567) (2.7156, -8.2487) (3.0395, -8.2487) knots 0 0 0 1 1 1
  line L1859 (2.4676, -8.0567) -> (2.7156, -8.2487) construction
  line L1860 (2.7156, -8.2487) -> (3.0395, -8.2487) construction
  line L1861 (3.0395, -8.2487) -> (3.2794, -8.2487)
  spline S539 degree 2 poles (3.2794, -8.2487) (3.5073, -8.2487) (3.6393, -8.0967) knots 0 0 0 1 1 1
  line L1862 (3.2794, -8.2487) -> (3.5073, -8.2487) construction
  line L1863 (3.5073, -8.2487) -> (3.6393, -8.0967) construction
  spline S540 degree 2 poles (3.6393, -8.0967) (3.7593, -7.9607) (3.7593, -7.7648) knots 0 0 0 1 1 1
  line L1864 (3.6393, -8.0967) -> (3.7593, -7.9607) construction
  line L1865 (3.7593, -7.9607) -> (3.7593, -7.7648) construction
  spline S541 degree 2 poles (3.7593, -7.7648) (3.7593, -7.3369) (3.3434, -7.2929) knots 0 0 0 1 1 1
  line L1866 (3.7593, -7.7648) -> (3.7593, -7.3369) construction
  line L1867 (3.7593, -7.3369) -> (3.3434, -7.2929) construction
  line L1868 (3.3434, -7.2929) -> (3.0435, -7.2929)
  spline S542 degree 2 poles (13.3366, -8.2487) (13.5325, -8.2487) (13.8124, -7.9647) (13.8124, -7.7688) knots 0 0 0 1 2 2 2
  line L1869 (13.3366, -8.2487) -> (13.5325, -8.2487) construction
  line L1870 (13.5325, -8.2487) -> (13.8124, -7.9647) construction
  line L1871 (13.8124, -7.9647) -> (13.8124, -7.7688) construction
  spline S543 degree 2 poles (12.8567, -5.8573) (12.6608, -5.8573) (12.3808, -6.1413) (12.3808, -6.3372) knots 0 0 0 1 2 2 2
  line L1872 (12.8567, -5.8573) -> (12.6608, -5.8573) construction
  line L1873 (12.6608, -5.8573) -> (12.3808, -6.1413) construction
  line L1874 (12.3808, -6.1413) -> (12.3808, -6.3372) construction
  line L1875 (12.3808, -6.3372) -> (12.3808, -7.7688)
  spline S544 degree 2 poles (12.3808, -7.7688) (12.3808, -7.9647) (12.6608, -8.2487) (12.8567, -8.2487) knots 0 0 0 1 2 2 2
  line L1876 (12.3808, -7.7688) -> (12.3808, -7.9647) construction
  line L1877 (12.3808, -7.9647) -> (12.6608, -8.2487) construction
  line L1878 (12.6608, -8.2487) -> (12.8567, -8.2487) construction
  line L1879 (12.8567, -8.2487) -> (13.3366, -8.2487)
  line L1880 (13.3366, -8.7285) -> (12.8567, -8.7285)
  spline S545 degree 2 poles (12.8567, -8.7285) (12.4648, -8.7285) (11.901, -8.1687) (11.901, -7.7728) knots 0 0 0 1 2 2 2
  line L1881 (12.8567, -8.7285) -> (12.4648, -8.7285) construction
  line L1882 (12.4648, -8.7285) -> (11.901, -8.1687) construction
  line L1883 (11.901, -8.1687) -> (11.901, -7.7728) construction
  line L1884 (11.901, -7.7728) -> (11.901, -6.3332)
  spline S546 degree 2 poles (11.901, -6.3332) (11.901, -5.9373) (12.4648, -5.3775) (12.8567, -5.3775) knots 0 0 0 1 2 2 2
  line L1885 (11.901, -6.3332) -> (11.901, -5.9373) construction
  line L1886 (11.901, -5.9373) -> (12.4648, -5.3775) construction
  line L1887 (12.4648, -5.3775) -> (12.8567, -5.3775) construction
  line L1888 (12.8567, -5.3775) -> (14.0524, -5.3775)
  spline S547 degree 2 poles (14.0524, -5.3775) (14.2923, -5.3775) (14.2923, -5.6174) knots 0 0 0 1 1 1
  line L1889 (14.0524, -5.3775) -> (14.2923, -5.3775) construction
  line L1890 (14.2923, -5.3775) -> (14.2923, -5.6174) construction
  line L1891 (14.2923, -5.6174) -> (14.2923, -7.7648)
  spline S548 degree 2 poles (14.2923, -7.7648) (14.2923, -8.1247) (14.6282, -8.2687) knots 0 0 0 1 1 1
  line L1892 (14.2923, -7.7648) -> (14.2923, -8.1247) construction
  line L1893 (14.2923, -8.1247) -> (14.6282, -8.2687) construction
  spline S549 degree 2 poles (14.6282, -8.2687) (14.7762, -8.3286) (14.7762, -8.4806) knots 0 0 0 1 1 1
  line L1894 (14.6282, -8.2687) -> (14.7762, -8.3286) construction
  line L1895 (14.7762, -8.3286) -> (14.7762, -8.4806) construction
  spline S550 degree 2 poles (14.7762, -8.4806) (14.7762, -8.5806) (14.6402, -8.7325) (14.5402, -8.7325) knots 0 0 0 1 2 2 2
  line L1896 (14.7762, -8.4806) -> (14.7762, -8.5806) construction
  line L1897 (14.7762, -8.5806) -> (14.6402, -8.7325) construction
  line L1898 (14.6402, -8.7325) -> (14.5402, -8.7325) construction
  spline S551 degree 2 poles (14.5402, -8.7325) (14.4883, -8.7325) (14.4363, -8.7085) knots 0 0 0 1 1 1
  line L1899 (14.5402, -8.7325) -> (14.4883, -8.7325) construction
  line L1900 (14.4883, -8.7325) -> (14.4363, -8.7085) construction
  spline S552 degree 2 poles (14.4363, -8.7085) (14.1963, -8.6046) (14.0484, -8.4126) knots 0 0 0 1 1 1
  line L1901 (14.4363, -8.7085) -> (14.1963, -8.6046) construction
  line L1902 (14.1963, -8.6046) -> (14.0484, -8.4126) construction
  spline S553 degree 2 poles (14.0484, -8.4126) (13.7605, -8.7285) (13.3366, -8.7285) knots 0 0 0 1 1 1
  line L1903 (14.0484, -8.4126) -> (13.7605, -8.7285) construction
  line L1904 (13.7605, -8.7285) -> (13.3366, -8.7285) construction
  spline S554 degree 2 poles (17.4034, -8.7285) (17.1635, -8.7285) (17.1635, -8.4886) knots 0 0 0 1 1 1
  line L1905 (17.4034, -8.7285) -> (17.1635, -8.7285) construction
  line L1906 (17.1635, -8.7285) -> (17.1635, -8.4886) construction
  spline S555 degree 2 poles (15.7159, -8.5646) (15.6639, -8.7285) (15.504, -8.7285) knots 0 0 0 1 1 1
  line L1907 (15.7159, -8.5646) -> (15.6639, -8.7285) construction
  line L1908 (15.6639, -8.7285) -> (15.504, -8.7285) construction
  spline S556 degree 2 poles (15.504, -8.7285) (15.252, -8.7285) (15.252, -8.5006) knots 0 0 0 1 1 1
  line L1909 (15.504, -8.7285) -> (15.252, -8.7285) construction
  line L1910 (15.252, -8.7285) -> (15.252, -8.5006) construction
  spline S557 degree 2 poles (15.252, -8.5006) (15.252, -8.4566) (15.268, -8.4126) knots 0 0 0 1 1 1
  line L1911 (15.252, -8.5006) -> (15.252, -8.4566) construction
  line L1912 (15.252, -8.4566) -> (15.268, -8.4126) construction
  line L1913 (15.268, -8.4126) -> (16.2158, -5.5414)
  spline S558 degree 2 poles (16.2158, -5.5414) (16.2677, -5.3775) (16.4397, -5.3775) knots 0 0 0 1 1 1
  line L1914 (16.2158, -5.5414) -> (16.2677, -5.3775) construction
  line L1915 (16.2677, -5.3775) -> (16.4397, -5.3775) construction
  line L1916 (16.4397, -5.3775) -> (17.4034, -5.3775)
  spline S559 degree 2 poles (17.4034, -5.3775) (17.6434, -5.3775) (17.6434, -5.6174) knots 0 0 0 1 1 1
  line L1917 (17.4034, -5.3775) -> (17.6434, -5.3775) construction
  line L1918 (17.6434, -5.3775) -> (17.6434, -5.6174) construction
  line L1919 (17.6434, -5.6174) -> (17.6434, -8.4886)
  spline S560 degree 2 poles (17.6434, -8.4886) (17.6434, -8.7285) (17.4034, -8.7285) knots 0 0 0 1 1 1
  line L1920 (17.6434, -8.4886) -> (17.6434, -8.7285) construction
  line L1921 (17.6434, -8.7285) -> (17.4034, -8.7285) construction
  spline S561 degree 2 poles (-20.1725, -22.1122) (-19.9765, -22.1122) (-19.6966, -21.8283) (-19.6966, -21.6323) knots 0 0 0 1 2 2 2
  line L1922 (-20.1725, -22.1122) -> (-19.9765, -22.1122) construction
  line L1923 (-19.9765, -22.1122) -> (-19.6966, -21.8283) construction
  line L1924 (-19.6966, -21.8283) -> (-19.6966, -21.6323) construction
  spline S562 degree 2 poles (-20.6523, -19.7209) (-20.8483, -19.7209) (-21.1282, -20.0048) (-21.1282, -20.2007) knots 0 0 0 1 2 2 2
  line L1925 (-20.6523, -19.7209) -> (-20.8483, -19.7209) construction
  line L1926 (-20.8483, -19.7209) -> (-21.1282, -20.0048) construction
  line L1927 (-21.1282, -20.0048) -> (-21.1282, -20.2007) construction
  line L1928 (-21.1282, -20.2007) -> (-21.1282, -21.6323)
  spline S563 degree 2 poles (-21.1282, -21.6323) (-21.1282, -21.8283) (-20.8483, -22.1122) (-20.6523, -22.1122) knots 0 0 0 1 2 2 2
  line L1929 (-21.1282, -21.6323) -> (-21.1282, -21.8283) construction
  line L1930 (-21.1282, -21.8283) -> (-20.8483, -22.1122) construction
  line L1931 (-20.8483, -22.1122) -> (-20.6523, -22.1122) construction
  line L1932 (-20.6523, -22.1122) -> (-20.1725, -22.1122)
  line L1933 (-20.1725, -22.5921) -> (-20.6523, -22.5921)
  spline S564 degree 2 poles (-20.6523, -22.5921) (-21.0442, -22.5921) (-21.6081, -22.0322) (-21.6081, -21.6363) knots 0 0 0 1 2 2 2
  line L1934 (-20.6523, -22.5921) -> (-21.0442, -22.5921) construction
  line L1935 (-21.0442, -22.5921) -> (-21.6081, -22.0322) construction
  line L1936 (-21.6081, -22.0322) -> (-21.6081, -21.6363) construction
  line L1937 (-21.6081, -21.6363) -> (-21.6081, -20.1967)
  spline S565 degree 2 poles (-21.6081, -20.1967) (-21.6081, -19.8008) (-21.0442, -19.241) (-20.6523, -19.241) knots 0 0 0 1 2 2 2
  line L1938 (-21.6081, -20.1967) -> (-21.6081, -19.8008) construction
  line L1939 (-21.6081, -19.8008) -> (-21.0442, -19.241) construction
  line L1940 (-21.0442, -19.241) -> (-20.6523, -19.241) construction
  line L1941 (-20.6523, -19.241) -> (-19.4567, -19.241)
  spline S566 degree 2 poles (-19.4567, -19.241) (-19.2167, -19.241) (-19.2167, -19.4809) knots 0 0 0 1 1 1
  line L1942 (-19.4567, -19.241) -> (-19.2167, -19.241) construction
  line L1943 (-19.2167, -19.241) -> (-19.2167, -19.4809) construction
  line L1944 (-19.2167, -19.4809) -> (-19.2167, -21.6283)
  spline S567 degree 2 poles (-19.2167, -21.6283) (-19.2167, -21.9882) (-18.8808, -22.1322) knots 0 0 0 1 1 1
  line L1945 (-19.2167, -21.6283) -> (-19.2167, -21.9882) construction
  line L1946 (-19.2167, -21.9882) -> (-18.8808, -22.1322) construction
  spline S568 degree 2 poles (-18.8808, -22.1322) (-18.7329, -22.1922) (-18.7329, -22.3441) knots 0 0 0 1 1 1
  line L1947 (-18.8808, -22.1322) -> (-18.7329, -22.1922) construction
  line L1948 (-18.7329, -22.1922) -> (-18.7329, -22.3441) construction
  spline S569 degree 2 poles (-18.7329, -22.3441) (-18.7329, -22.4441) (-18.8688, -22.5961) (-18.9688, -22.5961) knots 0 0 0 1 2 2 2
  line L1949 (-18.7329, -22.3441) -> (-18.7329, -22.4441) construction
  line L1950 (-18.7329, -22.4441) -> (-18.8688, -22.5961) construction
  line L1951 (-18.8688, -22.5961) -> (-18.9688, -22.5961) construction
  spline S570 degree 2 poles (-18.9688, -22.5961) (-19.0208, -22.5961) (-19.0728, -22.5721) knots 0 0 0 1 1 1
  line L1952 (-18.9688, -22.5961) -> (-19.0208, -22.5961) construction
  line L1953 (-19.0208, -22.5961) -> (-19.0728, -22.5721) construction
  spline S571 degree 2 poles (-19.0728, -22.5721) (-19.3127, -22.4681) (-19.4607, -22.2761) knots 0 0 0 1 1 1
  line L1954 (-19.0728, -22.5721) -> (-19.3127, -22.4681) construction
  line L1955 (-19.3127, -22.4681) -> (-19.4607, -22.2761) construction
  spline S572 degree 2 poles (-19.4607, -22.2761) (-19.7486, -22.5921) (-20.1725, -22.5921) knots 0 0 0 1 1 1
  line L1956 (-19.4607, -22.2761) -> (-19.7486, -22.5921) construction
  line L1957 (-19.7486, -22.5921) -> (-20.1725, -22.5921) construction
  spline S573 degree 2 poles (-16.1056, -22.5921) (-16.3456, -22.5921) (-16.3456, -22.3521) knots 0 0 0 1 1 1
  line L1958 (-16.1056, -22.5921) -> (-16.3456, -22.5921) construction
  line L1959 (-16.3456, -22.5921) -> (-16.3456, -22.3521) construction
  line L1960 (-16.3456, -22.3521) -> (-16.3456, -20.2007)
  spline S574 degree 2 poles (-16.3456, -20.2007) (-16.3456, -20.0048) (-16.6255, -19.7209) (-16.8214, -19.7209) knots 0 0 0 1 2 2 2
  line L1961 (-16.3456, -20.2007) -> (-16.3456, -20.0048) construction
  line L1962 (-16.3456, -20.0048) -> (-16.6255, -19.7209) construction
  line L1963 (-16.6255, -19.7209) -> (-16.8214, -19.7209) construction
  spline S575 degree 2 poles (-17.7771, -22.3521) (-17.7771, -22.5921) (-18.0171, -22.5921) knots 0 0 0 1 1 1
  line L1964 (-17.7771, -22.3521) -> (-17.7771, -22.5921) construction
  line L1965 (-17.7771, -22.5921) -> (-18.0171, -22.5921) construction
  spline S576 degree 2 poles (-18.0171, -22.5921) (-18.257, -22.5921) (-18.257, -22.3521) knots 0 0 0 1 1 1
  line L1966 (-18.0171, -22.5921) -> (-18.257, -22.5921) construction
  line L1967 (-18.257, -22.5921) -> (-18.257, -22.3521) construction
  line L1968 (-18.257, -22.3521) -> (-18.257, -19.4809)
  spline S577 degree 2 poles (-18.257, -19.4809) (-18.257, -19.241) (-18.0171, -19.241) knots 0 0 0 1 1 1
  line L1969 (-18.257, -19.4809) -> (-18.257, -19.241) construction
  line L1970 (-18.257, -19.241) -> (-18.0171, -19.241) construction
  line L1971 (-18.0171, -19.241) -> (-16.8214, -19.241)
  spline S578 degree 2 poles (-16.8214, -19.241) (-16.4255, -19.241) (-15.8657, -19.8008) (-15.8657, -20.1967) knots 0 0 0 1 2 2 2
  line L1972 (-16.8214, -19.241) -> (-16.4255, -19.241) construction
  line L1973 (-16.4255, -19.241) -> (-15.8657, -19.8008) construction
  line L1974 (-15.8657, -19.8008) -> (-15.8657, -20.1967) construction
  line L1975 (-15.8657, -20.1967) -> (-15.8657, -22.3521)
  spline S579 degree 2 poles (-15.8657, -22.3521) (-15.8657, -22.5921) (-16.1056, -22.5921) knots 0 0 0 1 1 1
  line L1976 (-15.8657, -22.3521) -> (-15.8657, -22.5921) construction
  line L1977 (-15.8657, -22.5921) -> (-16.1056, -22.5921) construction
  spline S580 degree 2 poles (-10.5952, -22.5921) (-10.9871, -22.5921) (-11.5549, -22.0322) (-11.5549, -21.6363) knots 0 0 0 1 2 2 2
  line L1978 (-10.5952, -22.5921) -> (-10.9871, -22.5921) construction
  line L1979 (-10.9871, -22.5921) -> (-11.5549, -22.0322) construction
  line L1980 (-11.5549, -22.0322) -> (-11.5549, -21.6363) construction
  line L1981 (-11.5549, -21.6363) -> (-11.5549, -20.1967)
  spline S581 degree 2 poles (-11.5549, -20.1967) (-11.5549, -19.8008) (-10.9871, -19.241) (-10.5952, -19.241) knots 0 0 0 1 2 2 2
  line L1982 (-11.5549, -20.1967) -> (-11.5549, -19.8008) construction
  line L1983 (-11.5549, -19.8008) -> (-10.9871, -19.241) construction
  line L1984 (-10.9871, -19.241) -> (-10.5952, -19.241) construction
  line L1985 (-10.5952, -19.241) -> (-9.8794, -19.241)
  spline S582 degree 2 poles (-9.8794, -19.241) (-9.6394, -19.241) (-9.6394, -19.4809) knots 0 0 0 1 1 1
  line L1986 (-9.8794, -19.241) -> (-9.6394, -19.241) construction
  line L1987 (-9.6394, -19.241) -> (-9.6394, -19.4809) construction
  spline S583 degree 2 poles (-9.6394, -19.4809) (-9.6394, -19.7209) (-9.8794, -19.7209) knots 0 0 0 1 1 1
  line L1988 (-9.6394, -19.4809) -> (-9.6394, -19.7209) construction
  line L1989 (-9.6394, -19.7209) -> (-9.8794, -19.7209) construction
  line L1990 (-9.8794, -19.7209) -> (-10.5952, -19.7209)
  spline S584 degree 2 poles (-10.5952, -19.7209) (-10.7911, -19.7209) (-11.075, -20.0048) (-11.075, -20.2007) knots 0 0 0 1 2 2 2
  line L1991 (-10.5952, -19.7209) -> (-10.7911, -19.7209) construction
  line L1992 (-10.7911, -19.7209) -> (-11.075, -20.0048) construction
  line L1993 (-11.075, -20.0048) -> (-11.075, -20.2007) construction
  line L1994 (-11.075, -20.2007) -> (-11.075, -21.6323)
  spline S585 degree 2 poles (-11.075, -21.6323) (-11.075, -21.8283) (-10.7911, -22.1122) (-10.5952, -22.1122) knots 0 0 0 1 2 2 2
  line L1995 (-11.075, -21.6323) -> (-11.075, -21.8283) construction
  line L1996 (-11.075, -21.8283) -> (-10.7911, -22.1122) construction
  line L1997 (-10.7911, -22.1122) -> (-10.5952, -22.1122) construction
  line L1998 (-10.5952, -22.1122) -> (-9.8794, -22.1122)
  spline S586 degree 2 poles (-9.8794, -22.1122) (-9.6394, -22.1122) (-9.6394, -22.3521) knots 0 0 0 1 1 1
  line L1999 (-9.8794, -22.1122) -> (-9.6394, -22.1122) construction